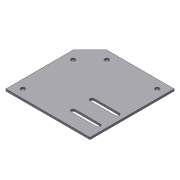
# Autodesk Inventor part: GearboxMountPlate
Saved by Autodesk Inventor 2012 (Build 160160000, 160)
## iProperties
Created: 2013-01-07
Part Number: GearboxMountPlate
Material: Aluminum-6061
Document SubType Name: Modeling
Designer: JesseK
Mass: 130.204 g
Surface Area: 326.946 cm^2
Volume: 48.0458 cm^3
Density: 2.71 g/cm^3
Author: JesseK
Autodesk Inventor part; units mm, degrees
ref_plane "YZ Plane" through (0, 0, 0) normal (1, 0, 0) x (0, 1, 0)
ref_plane "XZ Plane" through (0, 0, 0) normal (0, 1, 0) x (-1, 0, 0)
ref_plane "XY Plane" through (0, 0, 0) normal (0, 0, 1) x (1, 0, 0)
sketch "Sketch2" plane through (0, 0, 0) normal (0, 1, 0) x (-1, 0, 0)
  line L0 (0, 0) -> (0, 127)
  line L1 (0, 127) -> (127, 127)
  line L2 (127, 127) -> (127, 0)
  line L3 (127, 0) -> (0, 0)
  arc A0 (9.525, 107.95) -> (9.525, 101.6) centre (9.525, 104.775) ccw
  arc A1 (47.625, 101.6) -> (47.625, 107.95) centre (47.625, 104.775) ccw
  arc A2 (47.625, 73.025) -> (47.625, 79.375) centre (47.625, 76.2) ccw
  arc A3 (9.525, 79.375) -> (9.525, 73.025) centre (9.525, 76.2) ccw
  line L4 (9.525, 79.375) -> (47.625, 79.375)
  line L5 (47.625, 73.025) -> (9.525, 73.025)
  line L6 (9.525, 107.95) -> (47.625, 107.95)
  line L7 (47.625, 101.6) -> (9.525, 101.6)
  line L8 (9.525, 104.775) -> (9.525, 76.2) construction
  circle A4 centre (114.3, 114.3) radius 3.175
  circle A5 centre (114.3, 38.1) radius 3.175
  circle A6 centre (12.7, 12.7) radius 3.175
  circle A7 centre (88.9, 12.7) radius 3.175
  line L9 (114.3, 114.3) -> (114.3, 38.1) construction
  line L10 (12.7, 12.7) -> (88.9, 12.7) construction
  dimension "d7" = 127
  dimension "d18" = 38.1
  dimension "d19" = 79.375
  dimension "d22" = 12.7
  dimension "d23" = 76.2
  dimension "d24" = 76.2
  dimension "d25" = 6.35
  dimension "d28" = 12.7
  dimension "d29" = 12.7
  dimension "d30" = 38.1
  dimension "d31" = 127
  dimension "d32" = 9.525
  dimension "d36" = 12.7
  dimension "d39" = 22.225
  dimension "d40" = 28.575
  dimension "d41" = 76.2
  constraints: 22 end point, 8 centre point, 8 point on circle, 8 tangent, 7 horizontal, 5 equal radius, 4 vertical, 1 parallel
  measures "d7" distance of L0.start L0.end
  measures "d18" distance of L7.start L7.end
  measures "d19" distance from line of L2 A1.centre
  measures "d22" distance from line of L2 L9.end
  measures "d23" distance of L9.start L9.end
  measures "d24" distance of L10.start L10.end
  measures "d25" diameter of A5
  measures "d28" distance between parallel lines of L3 L10
  measures "d29" distance from line of L0 L10.start
  measures "d30" distance from line of L3 L9.end
  measures "d31" distance between parallel lines of L2 L0
  measures "d32" distance from line of L0 L8.start
  measures "d36" distance from line of L1 L9.start
  measures "d39" distance from line of L1 L8.start
  measures "d40" distance of L8.end L8.start
  measures "d41" distance from line of L3 L8.end
extrude "Extrusion3" add sketch "Sketch2" along normal blind 3.175
chamfer "Chamfer1" distance 25.4 angle 45 1 edges at (-127, 1.5875, 0)
body "Solid3"
